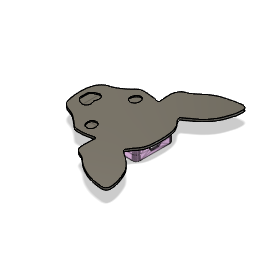
Case v4 (Autodesk Fusion 360 design; units mm, degrees)
Autodesk Fusion 360 part; units mm, degrees
mesh "Mesh1" [no effect]
sketch "Sketch1" plane through (0, 0, 0) normal (0, 1, 0) x (1, 0, 0)
  spline S0 degree 5 poles (79.7, 48.8) (79.719, 48.6987) (79.7514, 48.491) (79.7835, 48.1635) (79.7983, 47.6937) (79.7902, 47.047) (79.7751, 46.3439) (79.7599, 45.603) (79.7415, 44.8496) (79.7105, 44.1055) (79.6548, 43.3785) (79.5625, 42.6523) (79.4242, 41.8981) (79.2343, 41.0857) (78.9926, 40.1949) (78.7059, 39.2272) (78.3855, 38.1997) (78.0442, 37.1381) (77.6933, 36.0704) (77.3399, 35.0202) (76.9837, 33.9992) (76.6162, 33.0052) (76.2245, 32.0279) (75.7932, 31.0522) (75.3081, 30.0631) (74.7577, 29.0493) (74.1372, 28.0083) (73.4475, 26.9454) (72.6942, 25.8712) (71.8865, 24.8005) (71.0365, 23.75) (70.1577, 22.7363) (69.2645, 21.7746) (68.3706, 20.8762) (67.4886, 20.0487) (66.6282, 19.2945) (65.7956, 18.6106) (64.9922, 17.9877) (64.2136, 17.4094) (63.4483, 16.8517) (62.6821, 16.2893) (61.9016, 15.7016) (61.0986, 15.0793) (60.2738, 14.4301) (59.4412, 13.7868) (58.626, 13.1925) (57.8615, 12.684) (57.1871, 12.2757) (56.6448, 11.9441) (56.277, 11.6091) (56.116, 11.1755) (56.1708, 10.5839) (56.4188, 9.8471) (56.8189, 9.0183) (57.3225, 8.1658) (57.8852, 7.3451) (58.4778, 6.5734) (59.0828, 5.8405) (59.6904, 5.1182) (60.2951, 4.3704) (60.8923, 3.5627) (61.4748, 2.6725) (62.0334, 1.6874) (62.5584, 0.6036) (63.0405, -0.5757) (63.4715, -1.842) (63.846, -3.1831) (64.1621, -4.5843) (64.4206, -6.0301) (64.6252, -7.5046) (64.7808, -8.9924) (64.8936, -10.4799) (64.9703, -11.9557) (65.0169, -13.4121) (65.0389, -14.8453) (65.04, -16.2568) (65.0223, -17.6506) (64.9858, -19.0325) (64.9283, -20.4085) (64.8449, -21.783) (64.7281, -23.1575) (64.5673, -24.5293) (64.3484, -25.8898) (64.0567, -27.2263) (63.6793, -28.5249) (63.2076, -29.7715) (62.6403, -30.9546) (61.9852, -32.0673) (61.2629, -33.1089) (60.5082, -34.0874) (59.7625, -35.0146) (59.0668, -35.9023) (58.4531, -36.7574) (57.9381, -37.5785) (57.514, -38.3507) (57.1437, -39.0427) (56.7888, -39.6265) (56.4337, -40.094) (56.1169, -40.4782) (55.9432, -40.8613) (56.0142, -41.3227) (56.3554, -41.884) (56.9227, -42.515) (57.6412, -43.1657) (58.4327, -43.7883) (59.2513, -44.367) (60.0798, -44.9122) (60.9194, -45.4502) (61.7815, -46.0133) (62.6791, -46.6312) (63.617, -47.319) (64.5891, -48.0757) (65.5823, -48.8903) (66.5796, -49.7451) (67.5624, -50.6213) (68.5134, -51.5029) (69.4201, -52.3815) (70.2766, -53.2606) (71.083, -54.1521) (71.8431, -55.0725) (72.5629, -56.0393) (73.2493, -57.0672) (73.908, -58.165) (74.5421, -59.3304) (75.1517, -60.5514) (75.7351, -61.8097) (76.289, -63.0836) (76.8097, -64.3512) (77.294, -65.5936) (77.7391, -66.7979) (78.1445, -67.9606) (78.511, -69.0876) (78.84, -70.1896) (79.1328, -71.2793) (79.3893, -72.3679) (79.6075, -73.462) (79.7822, -74.5597) (79.9052, -75.6495) (79.9659, -76.714) (79.9523, -77.7308) (79.8515, -78.676) (79.651, -79.5255) (79.3392, -80.2577) (78.9071, -80.8561) (78.351, -81.3116) (77.674, -81.6255) (76.8884, -81.8117) (76.0116, -81.8922) (75.0626, -81.8922) (74.0586, -81.8357) (73.0105, -81.7401) (71.923, -81.6152) (70.7963, -81.4652) (69.6276, -81.2893) (68.413, -81.0833) (67.1491, -80.8408) (65.8342, -80.5541) (64.4698, -80.2157) (63.0597, -79.8186) (61.611, -79.3574) (60.1335, -78.8292) (58.6404, -78.2344) (57.148, -77.5774) (55.6761, -76.8675) (54.2482, -76.12) (52.889, -75.3539) (51.6218, -74.5894) (50.4661, -73.8459) (49.435, -73.1396) (48.5326, -72.4808) (47.752, -71.8723) (47.0713, -71.306) (46.4572, -70.7653) (45.8728, -70.232) (45.2832, -69.6907) (44.6638, -69.135) (44.0045, -68.5721) (43.3058, -68.0165) (42.5737, -67.4855) (41.8163, -66.994) (41.0385, -66.5495) (40.2417, -66.1497) (39.4275, -65.7856) (38.5995, -65.4415) (37.7661, -65.0972) (36.9437, -64.7285) (36.1534, -64.3102) (35.4181, -63.8185) (34.7592, -63.2338) (34.1931, -62.5432) (33.729, -61.7429) (33.3694, -60.8357) (33.1113, -59.8303) (32.9461, -58.7397) (32.8605, -57.58) (32.8372, -56.369) (32.8572, -55.1269) (32.9019, -53.8757) (32.9551, -52.6402) (33.0054, -51.4474) (33.0477, -50.327) (33.0862, -49.3112) (33.1287, -48.4278) (33.1813, -47.6907) (33.2433, -47.0941) (33.3012, -46.5995) (33.3258, -46.144) (33.2803, -45.6894) (33.1245, -45.2796) (32.838, -45.0016) (32.4755, -44.8703) (32.1398, -44.8181) (31.805, -44.8087) (31.3175, -44.855) (30.5696, -44.9693) (29.5634, -45.146) (28.365, -45.3694) (27.0805, -45.6165) (25.8227, -45.8622) (24.6834, -46.0835) (23.6982, -46.264) (22.8543, -46.3952) (22.1108, -46.4756) (21.4135, -46.5108) (20.7135, -46.5135) (19.9814, -46.5025) (19.2037, -46.4951) (18.3803, -46.5) (17.5215, -46.5088) (16.6451, -46.4914) (15.7717, -46.4081) (14.9204, -46.22) (14.1044, -45.8996) (13.3254, -45.4441) (12.575, -44.8733) (11.8395, -44.2198) (11.104, -43.5216) (10.3563, -42.8135) (9.5919, -42.1181) (8.8134, -41.4453) (8.0275, -40.7972) (7.2424, -40.1706) (6.4656, -39.5608) (5.7008, -38.9653) (4.9465, -38.3857) (4.1979, -37.8258) (3.4476, -37.291) (2.6872, -36.787) (1.9079, -36.3185) (1.1022, -35.8884) (0.2644, -35.4967) (-0.6087, -35.1391) (-1.5164, -34.807) (-2.4532, -34.4852) (-3.4094, -34.1535) (-4.3718, -33.7897) (-5.3247, -33.3723) (-6.2513, -32.8831) (-7.1342, -32.3101) (-7.9567, -31.6496) (-8.7041, -30.9033) (-9.3652, -30.0772) (-9.9331, -29.1799) (-10.4069, -28.2204) (-10.7931, -27.2066) (-11.1036, -26.1451) (-11.3536, -25.0408) (-11.5592, -23.8975) (-11.7349, -22.7174) (-11.8914, -21.5015) (-12.0333, -20.2492) (-12.16, -18.9596) (-12.2674, -17.6322) (-12.3489, -16.2679) (-12.3967, -14.8699) (-12.4034, -13.445) (-12.3627, -12.0041) (-12.2712, -10.5634) (-12.1273, -9.142) (-11.9309, -7.7602) (-11.6825, -6.4374) (-11.3825, -5.1897) (-11.0307, -4.0283) (-10.6255, -2.9572) (-10.1631, -1.971) (-9.6398, -1.0591) (-9.0533, -0.2097) (-8.4053, 0.5854) (-7.7029, 1.3276) (-6.9613, 2.0057) (-6.2025, 2.5971) (-5.4492, 3.0793) (-4.7184, 3.439) (-4.0167, 3.6808) (-3.3325, 3.8397) (-2.6411, 3.9728) (-1.9139, 4.1408) (-1.1273, 4.3941) (-0.2718, 4.7548) (0.6493, 5.2209) (1.6234, 5.7747) (2.6318, 6.39) (3.6529, 7.0395) (4.665, 7.7026) (5.6494, 8.3694) (6.5901, 9.0365) (7.4756, 9.7051) (8.2993, 10.3779) (9.0603, 11.0569) (9.7649, 11.7402) (10.4259, 12.4209) (11.0615, 13.0884) (11.6936, 13.7292) (12.3466, 14.3276) (13.0462, 14.8661) (13.8171, 15.3277) (14.6807, 15.6975) (15.6529, 15.9655) (16.7413, 16.1284) (17.9426, 16.1926) (19.243, 16.1724) (20.6205, 16.0873) (22.0464, 15.9583) (23.4868, 15.8057) (24.9046, 15.6459) (26.2614, 15.4886) (27.5183, 15.3328) (28.6412, 15.1715) (29.6053, 14.9976) (30.4017, 14.8101) (31.0401, 14.6197) (31.5593, 14.4564) (32.0179, 14.3687) (32.4563, 14.4031) (32.8494, 14.5822) (33.1244, 14.9053) (33.2471, 15.3733) (33.2474, 15.9939) (33.1791, 16.7718) (33.0898, 17.6996) (33.0018, 18.7535) (32.9234, 19.9011) (32.8536, 21.1057) (32.789, 22.3319) (32.7295, 23.5506) (32.6863, 24.7456) (32.6806, 25.9121) (32.738, 27.0512) (32.8842, 28.1659) (33.1401, 29.2558) (33.5175, 30.3134) (34.0136, 31.3181) (34.6121, 32.2394) (35.2891, 33.0464) (36.0178, 33.7154) (36.7729, 34.237) (37.5359, 34.6256) (38.2984, 34.9229) (39.0589, 35.1834) (39.8212, 35.4638) (40.5917, 35.8111) (41.378, 36.25) (42.1871, 36.7866) (43.0251, 37.4139) (43.896, 38.1159) (44.8012, 38.8726) (45.7384, 39.6653) (46.7022, 40.4774) (47.6866, 41.2944) (48.6859, 42.1039) (49.6968, 42.8958) (50.7197, 43.6621) (51.7606, 44.3973) (52.832, 45.098) (53.9494, 45.7628) (55.1293, 46.3915) (56.3853, 46.9846) (57.7261, 47.5433) (59.1523, 48.0682) (60.6535, 48.5596) (62.206, 49.0166) (63.7773, 49.4378) (65.3304, 49.8216) (66.8273, 50.1665) (68.2335, 50.4717) (69.5221, 50.7374) (70.6776, 50.9653) (71.7008, 51.1588) (72.6095, 51.3232) (73.4309, 51.4621) (74.1944, 51.5753) (74.925, 51.6566) (75.6357, 51.6895) (76.3257, 51.6523) (76.9846, 51.529) (77.5943, 51.3184) (78.1315, 51.0447) (78.5772, 50.7396) (78.926, 50.4252) (79.1962, 50.0932) (79.4146, 49.7205) (79.5553, 49.3789) (79.6375, 49.0986) (79.681, 48.9013) (79.7, 48.8) knots 0 0 0 0 0 0 0.0025 0.005 0.0075 0.01 0.0125 0.015 0.0175 0.02 0.0225 0.025 0.0275 0.03 0.0325 0.035 0.0375 0.04 0.0425 0.045 0.0475 0.05 0.0525 0.055 0.0575 0.06 0.0625 0.065 0.0675 0.07 0.0725 0.075 0.0775 0.08 0.0825 0.085 0.0875 0.09 0.0925 0.095 0.0975 0.1 0.1025 0.105 0.1075 0.11 0.1125 0.115 0.1175 0.12 0.1225 0.125 0.1275 0.13 0.1325 0.135 0.1375 0.14 0.1425 0.145 0.1475 0.15 0.1525 0.155 0.1575 0.16 0.1625 0.165 0.1675 0.17 0.1725 0.175 0.1775 0.18 0.1825 0.185 0.1875 0.19 0.1925 0.195 0.1975 0.2 0.2025 0.205 0.2075 0.21 0.2125 0.215 0.2175 0.22 0.2225 0.225 0.2275 0.23 0.2325 0.235 0.2375 0.24 0.2425 0.245 0.2475 0.25 0.2525 0.255 0.2575 0.26 0.2625 0.265 0.2675 0.27 0.2725 0.275 0.2775 0.28 0.2825 0.285 0.2875 0.29 0.2925 0.295 0.2975 0.3 0.3025 0.305 0.3075 0.31 0.3125 0.315 0.3175 0.32 0.3225 0.325 0.3275 0.33 0.3325 0.335 0.3375 0.34 0.3425 0.345 0.3475 0.35 0.3525 0.355 0.3575 0.36 0.3625 0.365 0.3675 0.37 0.3725 0.375 0.3775 0.38 0.3825 0.385 0.3875 0.39 0.3925 0.395 0.3975 0.4 0.4025 0.405 0.4075 0.41 0.4125 0.415 0.4175 0.42 0.4225 0.425 0.4275 0.43 0.4325 0.435 0.4375 0.44 0.4425 0.445 0.4475 0.45 0.4525 0.455 0.4575 0.46 0.4625 0.465 0.4675 0.47 0.4725 0.475 0.4775 0.48 0.4825 0.485 0.4875 0.49 0.4925 0.495 0.4975 0.5 0.5025 0.505 0.5075 0.51 0.5125 0.515 0.5175 0.52 0.5225 0.525 0.5275 0.53 0.5325 0.535 0.5375 0.54 0.5425 0.545 0.5475 0.55 0.5525 0.555 0.5575 0.56 0.5625 0.565 0.5675 0.57 0.5725 0.575 0.5775 0.58 0.5825 0.585 0.5875 0.59 0.5925 0.595 0.5975 0.6 0.6025 0.605 0.6075 0.61 0.6125 0.615 0.6175 0.62 0.6225 0.625 0.6275 0.63 0.6325 0.635 0.6375 0.64 0.6425 0.645 0.6475 0.65 0.6525 0.655 0.6575 0.66 0.6625 0.665 0.6675 0.67 0.6725 0.675 0.6775 0.68 0.6825 0.685 0.6875 0.69 0.6925 0.695 0.6975 0.7 0.7025 0.705 0.7075 0.71 0.7125 0.715 0.7175 0.72 0.7225 0.725 0.7275 0.73 0.7325 0.735 0.7375 0.74 0.7425 0.745 0.7475 0.75 0.7525 0.755 0.7575 0.76 0.7625 0.765 0.7675 0.77 0.7725 0.775 0.7775 0.78 0.7825 0.785 0.7875 0.79 0.7925 0.795 0.7975 0.8 0.8025 0.805 0.8075 0.81 0.8125 0.815 0.8175 0.82 0.8225 0.825 0.8275 0.83 0.8325 0.835 0.8375 0.84 0.8425 0.845 0.8475 0.85 0.8525 0.855 0.8575 0.86 0.8625 0.865 0.8675 0.87 0.8725 0.875 0.8775 0.88 0.8825 0.885 0.8875 0.89 0.8925 0.895 0.8975 0.9 0.9025 0.905 0.9075 0.91 0.9125 0.915 0.9175 0.92 0.9225 0.925 0.9275 0.93 0.9325 0.935 0.9375 0.94 0.9425 0.945 0.9475 0.95 0.9525 0.955 0.9575 0.96 0.9625 0.965 0.9675 0.97 0.9725 0.975 0.9775 0.98 0.9825 0.985 0.9875 0.99 0.9925 0.995 0.9975 1 1 1 1 1 1
  point P0 (79.7869, 46.9408)
  point P1 (79.7048, 44.1167)
  point P2 (79.2122, 41.0299)
  point P3 (77.5, 35.5)
  point P4 (75.193, 29.8677)
  point P5 (70.2659, 22.8745)
  point P6 (65, 18)
  point P7 (61, 15)
  point P8 (57.1735, 12.2655)
  point P9 (56.1802, 11.2125)
  point P10 (57.3126, 8.2126)
  point P11 (60.2997, 4.347)
  point P12 (63.5, -2)
  point P13 (65, -13)
  point P14 (64.7162, -23.1652)
  point P15 (62, -32)
  point P16 (58, -37.5)
  point P17 (56.5, -40)
  point P18 (56, -41)
  point P19 (57.7878, -43.2659)
  point P20 (62.2077, -46.3112)
  point P21 (68.5, -51.5)
  point P22 (73.5, -57.5)
  point P23 (77.4744, -66.0904)
  point P24 (79.5, -72.9496)
  point P25 (79.8271, -78.649)
  point P26 (78.336, -81.2667)
  point P27 (74.6579, -81.8632)
  point P28 (68, -81)
  point P29 (57.0626, -77.5224)
  point P30 (48.2484, -72.2537)
  point P31 (45.3656, -69.7685)
  point P32 (42.2508, -67.2833)
  point P33 (38.5097, -65.4045)
  point P34 (34.9376, -63.3633)
  point P35 (33, -59)
  point P36 (33.0058, -51.4078)
  point P37 (33.2245, -47.289)
  point P38 (33.3, -46)
  point P39 (32.9569, -45.1468)
  point P40 (32.3074, -44.8515)
  point P41 (31.466, -44.8466)
  point P42 (25.5907, -45.9068)
  point P43 (21.5, -46.5)
  point P44 (18.5, -46.5)
  point P45 (14.6259, -46.0847)
  point P46 (10.8622, -43.2937)
  point P47 (6.7439, -39.7801)
  point P48 (3, -37)
  point P49 (-1, -35)
  point P50 (-6, -33)
  point P51 (-10, -29)
  point P52 (-11.7363, -22.6636)
  point P53 (-12.3921, -13.4829)
  point P54 (-11, -4)
  point P55 (-8, 1)
  point P56 (-4.5, 3.5)
  point P57 (-1.7755, 4.1976)
  point P58 (3.2385, 6.7787)
  point P59 (8.6974, 10.7403)
  point P60 (12, 14)
  point P61 (16, 16)
  point P62 (25.2363, 15.6066)
  point P63 (30.8294, 14.6801)
  point P64 (32.2, 14.4)
  point P65 (33, 14.8)
  point P66 (33.2, 16.5)
  point P67 (32.769, 22.762)
  point P68 (33.2893, 29.6228)
  point P69 (36.5734, 34.0774)
  point P70 (39.89, 35.5081)
  point P71 (44.117, 38.3045)
  point P72 (50.5226, 43.507)
  point P73 (59, 48)
  point P74 (70.2921, 50.888)
  point P75 (74.4866, 51.6033)
  point P76 (77, 51.5)
  point P77 (78.6, 50.7)
  point P78 (79.3, 49.9)
extrude "Extrude1" add sketch "Sketch1" along normal blind 2 from surface at 17
sketch "Sketch2" plane through (0, 19, 0) normal (0, 1, 0) x (-1, 0, 0)
  spline S0 degree 5 poles (-79.7, -48.8) (-79.681, -48.9013) (-79.6375, -49.0986) (-79.5553, -49.3789) (-79.4146, -49.7205) (-79.1962, -50.0932) (-78.926, -50.4252) (-78.5772, -50.7396) (-78.1315, -51.0447) (-77.5943, -51.3184) (-76.9846, -51.529) (-76.3257, -51.6523) (-75.6357, -51.6895) (-74.925, -51.6566) (-74.1944, -51.5753) (-73.4309, -51.4621) (-72.6095, -51.3232) (-71.7008, -51.1588) (-70.6776, -50.9653) (-69.5221, -50.7374) (-68.2335, -50.4717) (-66.8273, -50.1665) (-65.3304, -49.8216) (-63.7773, -49.4378) (-62.206, -49.0166) (-60.6535, -48.5596) (-59.1523, -48.0682) (-57.7261, -47.5433) (-56.3853, -46.9846) (-55.1293, -46.3915) (-53.9494, -45.7628) (-52.832, -45.098) (-51.7606, -44.3973) (-50.7197, -43.6621) (-49.6968, -42.8958) (-48.6859, -42.1039) (-47.6866, -41.2944) (-46.7022, -40.4774) (-45.7384, -39.6653) (-44.8012, -38.8726) (-43.896, -38.1159) (-43.0251, -37.4139) (-42.1871, -36.7866) (-41.378, -36.25) (-40.5917, -35.8111) (-39.8212, -35.4638) (-39.0589, -35.1834) (-38.2984, -34.9229) (-37.5359, -34.6256) (-36.7729, -34.237) (-36.0178, -33.7154) (-35.2891, -33.0464) (-34.6121, -32.2394) (-34.0136, -31.3181) (-33.5175, -30.3134) (-33.1401, -29.2558) (-32.8842, -28.1659) (-32.738, -27.0512) (-32.6806, -25.9121) (-32.6863, -24.7456) (-32.7295, -23.5506) (-32.789, -22.3319) (-32.8536, -21.1057) (-32.9234, -19.9011) (-33.0018, -18.7535) (-33.0898, -17.6996) (-33.1791, -16.7718) (-33.2474, -15.9939) (-33.2471, -15.3733) (-33.1244, -14.9053) (-32.8494, -14.5822) (-32.4563, -14.4031) (-32.0179, -14.3687) (-31.5593, -14.4564) (-31.0401, -14.6197) (-30.4017, -14.8101) (-29.6053, -14.9976) (-28.6412, -15.1715) (-27.5183, -15.3328) (-26.2614, -15.4886) (-24.9046, -15.6459) (-23.4868, -15.8057) (-22.0464, -15.9583) (-20.6205, -16.0873) (-19.243, -16.1724) (-17.9426, -16.1926) (-16.7413, -16.1284) (-15.6529, -15.9655) (-14.6807, -15.6975) (-13.8171, -15.3277) (-13.0462, -14.8661) (-12.3466, -14.3276) (-11.6936, -13.7292) (-11.0615, -13.0884) (-10.4259, -12.4209) (-9.7649, -11.7402) (-9.0603, -11.0569) (-8.2993, -10.3779) (-7.4756, -9.7051) (-6.5901, -9.0365) (-5.6494, -8.3694) (-4.665, -7.7026) (-3.6529, -7.0395) (-2.6318, -6.39) (-1.6234, -5.7747) (-0.6493, -5.2209) (0.2718, -4.7548) (1.1273, -4.3941) (1.9139, -4.1408) (2.6411, -3.9728) (3.3325, -3.8397) (4.0167, -3.6808) (4.7184, -3.439) (5.4492, -3.0793) (6.2025, -2.5971) (6.9613, -2.0057) (7.7029, -1.3276) (8.4053, -0.5854) (9.0533, 0.2097) (9.6398, 1.0591) (10.1631, 1.971) (10.6255, 2.9572) (11.0307, 4.0283) (11.3825, 5.1897) (11.6825, 6.4374) (11.9309, 7.7602) (12.1273, 9.142) (12.2712, 10.5634) (12.3627, 12.0041) (12.4034, 13.445) (12.3967, 14.8699) (12.3489, 16.2679) (12.2674, 17.6322) (12.16, 18.9596) (12.0333, 20.2492) (11.8914, 21.5015) (11.7349, 22.7174) (11.5592, 23.8975) (11.3536, 25.0408) (11.1036, 26.1451) (10.7931, 27.2066) (10.4069, 28.2204) (9.9331, 29.1799) (9.3652, 30.0772) (8.7041, 30.9033) (7.9567, 31.6496) (7.1342, 32.3101) (6.2513, 32.8831) (5.3247, 33.3723) (4.3718, 33.7897) (3.4094, 34.1535) (2.4532, 34.4852) (1.5164, 34.807) (0.6087, 35.1391) (-0.2644, 35.4967) (-1.1022, 35.8884) (-1.9079, 36.3185) (-2.6872, 36.787) (-3.4476, 37.291) (-4.1979, 37.8258) (-4.9465, 38.3857) (-5.7008, 38.9653) (-6.4656, 39.5608) (-7.2424, 40.1706) (-8.0275, 40.7972) (-8.8134, 41.4453) (-9.5919, 42.1181) (-10.3563, 42.8135) (-11.104, 43.5216) (-11.8395, 44.2198) (-12.575, 44.8733) (-13.3254, 45.4441) (-14.1044, 45.8996) (-14.9204, 46.22) (-15.7717, 46.4081) (-16.6451, 46.4914) (-17.5215, 46.5088) (-18.3803, 46.5) (-19.2037, 46.4951) (-19.9814, 46.5025) (-20.7135, 46.5135) (-21.4135, 46.5108) (-22.1108, 46.4756) (-22.8543, 46.3952) (-23.6982, 46.264) (-24.6834, 46.0835) (-25.8227, 45.8622) (-27.0805, 45.6165) (-28.365, 45.3694) (-29.5634, 45.146) (-30.5696, 44.9693) (-31.3175, 44.855) (-31.805, 44.8087) (-32.1398, 44.8181) (-32.4755, 44.8703) (-32.838, 45.0016) (-33.1245, 45.2796) (-33.2803, 45.6894) (-33.3258, 46.144) (-33.3012, 46.5995) (-33.2433, 47.0941) (-33.1813, 47.6907) (-33.1287, 48.4278) (-33.0862, 49.3112) (-33.0477, 50.327) (-33.0054, 51.4474) (-32.9551, 52.6402) (-32.9019, 53.8757) (-32.8572, 55.1269) (-32.8372, 56.369) (-32.8605, 57.58) (-32.9461, 58.7397) (-33.1113, 59.8303) (-33.3694, 60.8357) (-33.729, 61.7429) (-34.1931, 62.5432) (-34.7592, 63.2338) (-35.4181, 63.8185) (-36.1534, 64.3102) (-36.9437, 64.7285) (-37.7661, 65.0972) (-38.5995, 65.4415) (-39.4275, 65.7856) (-40.2417, 66.1497) (-41.0385, 66.5495) (-41.8163, 66.994) (-42.5737, 67.4855) (-43.3058, 68.0165) (-44.0045, 68.5721) (-44.6638, 69.135) (-45.2832, 69.6907) (-45.8728, 70.232) (-46.4572, 70.7653) (-47.0713, 71.306) (-47.752, 71.8723) (-48.5326, 72.4808) (-49.435, 73.1396) (-50.4661, 73.8459) (-51.6218, 74.5894) (-52.889, 75.3539) (-54.2482, 76.12) (-55.6761, 76.8675) (-57.148, 77.5774) (-58.6404, 78.2344) (-60.1335, 78.8292) (-61.611, 79.3574) (-63.0597, 79.8186) (-64.4698, 80.2157) (-65.8342, 80.5541) (-67.1491, 80.8408) (-68.413, 81.0833) (-69.6276, 81.2893) (-70.7963, 81.4652) (-71.923, 81.6152) (-73.0105, 81.7401) (-74.0586, 81.8357) (-75.0626, 81.8922) (-76.0116, 81.8922) (-76.8884, 81.8117) (-77.674, 81.6255) (-78.351, 81.3116) (-78.9071, 80.8561) (-79.3392, 80.2577) (-79.651, 79.5255) (-79.8515, 78.676) (-79.9523, 77.7308) (-79.9659, 76.714) (-79.9052, 75.6495) (-79.7822, 74.5597) (-79.6075, 73.462) (-79.3893, 72.3679) (-79.1328, 71.2793) (-78.84, 70.1896) (-78.511, 69.0876) (-78.1445, 67.9606) (-77.7391, 66.7979) (-77.294, 65.5936) (-76.8097, 64.3512) (-76.289, 63.0836) (-75.7351, 61.8097) (-75.1517, 60.5514) (-74.5421, 59.3304) (-73.908, 58.165) (-73.2493, 57.0672) (-72.5629, 56.0393) (-71.8431, 55.0725) (-71.083, 54.1521) (-70.2766, 53.2606) (-69.4201, 52.3815) (-68.5134, 51.5029) (-67.5624, 50.6213) (-66.5796, 49.7451) (-65.5823, 48.8903) (-64.5891, 48.0757) (-63.617, 47.319) (-62.6791, 46.6312) (-61.7815, 46.0133) (-60.9194, 45.4502) (-60.0798, 44.9122) (-59.2513, 44.367) (-58.4327, 43.7883) (-57.6412, 43.1657) (-56.9227, 42.515) (-56.3554, 41.884) (-56.0142, 41.3227) (-55.9432, 40.8613) (-56.1169, 40.4782) (-56.4337, 40.094) (-56.7888, 39.6265) (-57.1437, 39.0427) (-57.514, 38.3507) (-57.9381, 37.5785) (-58.4531, 36.7574) (-59.0668, 35.9023) (-59.7625, 35.0146) (-60.5082, 34.0874) (-61.2629, 33.1089) (-61.9852, 32.0673) (-62.6403, 30.9546) (-63.2076, 29.7715) (-63.6793, 28.5249) (-64.0567, 27.2263) (-64.3484, 25.8898) (-64.5673, 24.5293) (-64.7281, 23.1575) (-64.8449, 21.783) (-64.9283, 20.4085) (-64.9858, 19.0325) (-65.0223, 17.6506) (-65.04, 16.2568) (-65.0389, 14.8453) (-65.0169, 13.4121) (-64.9703, 11.9557) (-64.8936, 10.4799) (-64.7808, 8.9924) (-64.6252, 7.5046) (-64.4206, 6.0301) (-64.1621, 4.5843) (-63.846, 3.1831) (-63.4715, 1.842) (-63.0405, 0.5757) (-62.5584, -0.6036) (-62.0334, -1.6874) (-61.4748, -2.6725) (-60.8923, -3.5627) (-60.2951, -4.3704) (-59.6904, -5.1182) (-59.0828, -5.8405) (-58.4778, -6.5734) (-57.8852, -7.3451) (-57.3225, -8.1658) (-56.8189, -9.0183) (-56.4188, -9.8471) (-56.1708, -10.5839) (-56.116, -11.1755) (-56.277, -11.6091) (-56.6448, -11.9441) (-57.1871, -12.2757) (-57.8615, -12.684) (-58.626, -13.1925) (-59.4412, -13.7868) (-60.2738, -14.4301) (-61.0986, -15.0793) (-61.9016, -15.7016) (-62.6821, -16.2893) (-63.4483, -16.8517) (-64.2136, -17.4094) (-64.9922, -17.9877) (-65.7956, -18.6106) (-66.6282, -19.2945) (-67.4886, -20.0487) (-68.3706, -20.8762) (-69.2645, -21.7746) (-70.1577, -22.7363) (-71.0365, -23.75) (-71.8865, -24.8005) (-72.6942, -25.8712) (-73.4475, -26.9454) (-74.1372, -28.0083) (-74.7577, -29.0493) (-75.3081, -30.0631) (-75.7932, -31.0522) (-76.2245, -32.0279) (-76.6162, -33.0052) (-76.9837, -33.9992) (-77.3399, -35.0202) (-77.6933, -36.0704) (-78.0442, -37.1381) (-78.3855, -38.1997) (-78.7059, -39.2272) (-78.9926, -40.1949) (-79.2343, -41.0857) (-79.4242, -41.8981) (-79.5625, -42.6523) (-79.6548, -43.3785) (-79.7105, -44.1055) (-79.7415, -44.8496) (-79.7599, -45.603) (-79.7751, -46.3439) (-79.7902, -47.047) (-79.7983, -47.6937) (-79.7835, -48.1635) (-79.7514, -48.491) (-79.719, -48.6987) (-79.7, -48.8) knots -1 -1 -1 -1 -1 -1 -0.9975 -0.995 -0.9925 -0.99 -0.9875 -0.985 -0.9825 -0.98 -0.9775 -0.975 -0.9725 -0.97 -0.9675 -0.965 -0.9625 -0.96 -0.9575 -0.955 -0.9525 -0.95 -0.9475 -0.945 -0.9425 -0.94 -0.9375 -0.935 -0.9325 -0.93 -0.9275 -0.925 -0.9225 -0.92 -0.9175 -0.915 -0.9125 -0.91 -0.9075 -0.905 -0.9025 -0.9 -0.8975 -0.895 -0.8925 -0.89 -0.8875 -0.885 -0.8825 -0.88 -0.8775 -0.875 -0.8725 -0.87 -0.8675 -0.865 -0.8625 -0.86 -0.8575 -0.855 -0.8525 -0.85 -0.8475 -0.845 -0.8425 -0.84 -0.8375 -0.835 -0.8325 -0.83 -0.8275 -0.825 -0.8225 -0.82 -0.8175 -0.815 -0.8125 -0.81 -0.8075 -0.805 -0.8025 -0.8 -0.7975 -0.795 -0.7925 -0.79 -0.7875 -0.785 -0.7825 -0.78 -0.7775 -0.775 -0.7725 -0.77 -0.7675 -0.765 -0.7625 -0.76 -0.7575 -0.755 -0.7525 -0.75 -0.7475 -0.745 -0.7425 -0.74 -0.7375 -0.735 -0.7325 -0.73 -0.7275 -0.725 -0.7225 -0.72 -0.7175 -0.715 -0.7125 -0.71 -0.7075 -0.705 -0.7025 -0.7 -0.6975 -0.695 -0.6925 -0.69 -0.6875 -0.685 -0.6825 -0.68 -0.6775 -0.675 -0.6725 -0.67 -0.6675 -0.665 -0.6625 -0.66 -0.6575 -0.655 -0.6525 -0.65 -0.6475 -0.645 -0.6425 -0.64 -0.6375 -0.635 -0.6325 -0.63 -0.6275 -0.625 -0.6225 -0.62 -0.6175 -0.615 -0.6125 -0.61 -0.6075 -0.605 -0.6025 -0.6 -0.5975 -0.595 -0.5925 -0.59 -0.5875 -0.585 -0.5825 -0.58 -0.5775 -0.575 -0.5725 -0.57 -0.5675 -0.565 -0.5625 -0.56 -0.5575 -0.555 -0.5525 -0.55 -0.5475 -0.545 -0.5425 -0.54 -0.5375 -0.535 -0.5325 -0.53 -0.5275 -0.525 -0.5225 -0.52 -0.5175 -0.515 -0.5125 -0.51 -0.5075 -0.505 -0.5025 -0.5 -0.4975 -0.495 -0.4925 -0.49 -0.4875 -0.485 -0.4825 -0.48 -0.4775 -0.475 -0.4725 -0.47 -0.4675 -0.465 -0.4625 -0.46 -0.4575 -0.455 -0.4525 -0.45 -0.4475 -0.445 -0.4425 -0.44 -0.4375 -0.435 -0.4325 -0.43 -0.4275 -0.425 -0.4225 -0.42 -0.4175 -0.415 -0.4125 -0.41 -0.4075 -0.405 -0.4025 -0.4 -0.3975 -0.395 -0.3925 -0.39 -0.3875 -0.385 -0.3825 -0.38 -0.3775 -0.375 -0.3725 -0.37 -0.3675 -0.365 -0.3625 -0.36 -0.3575 -0.355 -0.3525 -0.35 -0.3475 -0.345 -0.3425 -0.34 -0.3375 -0.335 -0.3325 -0.33 -0.3275 -0.325 -0.3225 -0.32 -0.3175 -0.315 -0.3125 -0.31 -0.3075 -0.305 -0.3025 -0.3 -0.2975 -0.295 -0.2925 -0.29 -0.2875 -0.285 -0.2825 -0.28 -0.2775 -0.275 -0.2725 -0.27 -0.2675 -0.265 -0.2625 -0.26 -0.2575 -0.255 -0.2525 -0.25 -0.2475 -0.245 -0.2425 -0.24 -0.2375 -0.235 -0.2325 -0.23 -0.2275 -0.225 -0.2225 -0.22 -0.2175 -0.215 -0.2125 -0.21 -0.2075 -0.205 -0.2025 -0.2 -0.1975 -0.195 -0.1925 -0.19 -0.1875 -0.185 -0.1825 -0.18 -0.1775 -0.175 -0.1725 -0.17 -0.1675 -0.165 -0.1625 -0.16 -0.1575 -0.155 -0.1525 -0.15 -0.1475 -0.145 -0.1425 -0.14 -0.1375 -0.135 -0.1325 -0.13 -0.1275 -0.125 -0.1225 -0.12 -0.1175 -0.115 -0.1125 -0.11 -0.1075 -0.105 -0.1025 -0.1 -0.0975 -0.095 -0.0925 -0.09 -0.0875 -0.085 -0.0825 -0.08 -0.0775 -0.075 -0.0725 -0.07 -0.0675 -0.065 -0.0625 -0.06 -0.0575 -0.055 -0.0525 -0.05 -0.0475 -0.045 -0.0425 -0.04 -0.0375 -0.035 -0.0325 -0.03 -0.0275 -0.025 -0.0225 -0.02 -0.0175 -0.015 -0.0125 -0.01 -0.0075 -0.005 -0.0025 0 0 0 0 0 0
  spline S1 degree 5 poles (-21.9, 31.6) (-21.9594, 31.6337) (-22.0768, 31.7044) (-22.2495, 31.8196) (-22.4754, 31.991) (-22.748, 32.2339) (-23.0047, 32.5042) (-23.24, 32.7995) (-23.4516, 33.117) (-23.6388, 33.4551) (-23.8022, 33.8155) (-23.9429, 34.205) (-24.0616, 34.6344) (-24.1576, 35.1137) (-24.2276, 35.6486) (-24.2643, 36.2363) (-24.2563, 36.8627) (-24.1902, 37.5067) (-24.0527, 38.1431) (-23.8329, 38.7459) (-23.5245, 39.2917) (-23.1279, 39.7632) (-22.6508, 40.1499) (-22.1056, 40.4459) (-21.5086, 40.6485) (-20.8779, 40.7571) (-20.2323, 40.7707) (-19.5893, 40.6877) (-18.9654, 40.5061) (-18.3753, 40.2248) (-17.8319, 39.8452) (-17.3457, 39.3713) (-16.9248, 38.8118) (-16.5744, 38.18) (-16.298, 37.4928) (-16.0979, 36.7694) (-15.9759, 36.0302) (-15.9344, 35.2961) (-15.9763, 34.5865) (-16.1068, 33.9192) (-16.3307, 33.3091) (-16.6506, 32.7684) (-17.0644, 32.3059) (-17.563, 31.9269) (-18.1282, 31.6325) (-18.7308, 31.4196) (-19.3371, 31.282) (-19.9141, 31.2118) (-20.4352, 31.2001) (-20.8855, 31.2384) (-21.2685, 31.3197) (-21.5343, 31.4151) (-21.7203, 31.5019) (-21.8406, 31.5663) (-21.9, 31.6) knots 0 0 0 0 0 0 0.02 0.04 0.06 0.08 0.1 0.12 0.14 0.16 0.18 0.2 0.22 0.24 0.26 0.28 0.3 0.32 0.34 0.36 0.38 0.4 0.42 0.44 0.46 0.48 0.5 0.52 0.54 0.56 0.58 0.6 0.62 0.64 0.66 0.68 0.7 0.72 0.74 0.76 0.78 0.8 0.82 0.84 0.86 0.88 0.9 0.92 0.94 0.96 0.98 1 1 1 1 1 1
  spline S2 degree 5 poles (-23.5098, -8.5144) (-23.5711, -8.4113) (-23.6861, -8.2053) (-23.8364, -7.8978) (-23.9955, -7.4925) (-24.1361, -6.9835) (-24.2278, -6.4565) (-24.2746, -5.8972) (-24.2708, -5.3011) (-24.203, -4.6731) (-24.055, -4.0256) (-23.8113, -3.377) (-23.4611, -2.7501) (-23.0012, -2.1707) (-22.4358, -1.665) (-21.7761, -1.2585) (-21.0401, -0.9732) (-20.2528, -0.8259) (-19.4458, -0.8263) (-18.6543, -0.9769) (-17.914, -1.274) (-17.2579, -1.7079) (-16.7133, -2.2631) (-16.2978, -2.919) (-16.0191, -3.6506) (-15.8773, -4.431) (-15.8667, -5.2333) (-15.9779, -6.0324) (-16.1995, -6.8072) (-16.5204, -7.5423) (-16.929, -8.2261) (-17.4132, -8.8489) (-17.9602, -9.4002) (-18.5564, -9.8674) (-19.1867, -10.2328) (-19.8348, -10.4748) (-20.484, -10.5744) (-21.1172, -10.5197) (-21.7182, -10.3115) (-22.2716, -9.9697) (-22.7638, -9.5298) (-23.1005, -9.1316) (-23.3185, -8.8236) (-23.4486, -8.6174) (-23.5098, -8.5144) knots 0 0 0 0 0 0 0.025 0.05 0.075 0.1 0.125 0.15 0.175 0.2 0.225 0.25 0.275 0.3 0.325 0.35 0.375 0.4 0.425 0.45 0.475 0.5 0.525 0.55 0.575 0.6 0.625 0.65 0.675 0.7 0.725 0.75 0.775 0.8 0.825 0.85 0.875 0.9 0.925 0.95 0.975 1 1 1 1 1 1
  spline S3 degree 5 poles (7.7509, 15.4792) (7.7463, 15.3221) (7.7417, 15.0047) (7.7496, 14.5195) (7.7839, 13.8566) (7.8253, 13.0186) (7.8096, 12.1943) (7.6819, 11.4079) (7.4001, 10.6803) (6.9519, 10.0235) (6.3583, 9.4392) (5.6599, 8.9232) (4.9077, 8.4683) (4.1512, 8.0677) (3.4294, 7.7179) (2.7576, 7.4228) (2.1321, 7.1923) (1.5389, 7.0385) (0.9612, 6.9741) (0.387, 7.0089) (-0.1833, 7.1476) (-0.7403, 7.3909) (-1.2679, 7.7361) (-1.7466, 8.1784) (-2.1556, 8.7117) (-2.476, 9.3274) (-2.6935, 10.0133) (-2.8012, 10.7525) (-2.8025, 11.5212) (-2.7135, 12.2889) (-2.5593, 13.0242) (-2.371, 13.7005) (-2.1831, 14.3021) (-2.0297, 14.8298) (-1.942, 15.3055) (-1.9416, 15.7608) (-2.0354, 16.2269) (-2.2078, 16.7226) (-2.4228, 17.2519) (-2.6356, 17.8113) (-2.8018, 18.3949) (-2.889, 19.0012) (-2.8796, 19.6335) (-2.7646, 20.2932) (-2.5396, 20.9739) (-2.1998, 21.6562) (-1.735, 22.3015) (-1.135, 22.8604) (-0.3933, 23.2809) (0.487, 23.5172) (1.4893, 23.5377) (2.5772, 23.3352) (3.6958, 22.9278) (4.7815, 22.3504) (5.7696, 21.6483) (6.6022, 20.8706) (7.2364, 20.0633) (7.652, 19.2629) (7.8612, 18.4886) (7.9106, 17.7391) (7.864, 17.0013) (7.8034, 16.4054) (7.7693, 15.9476) (7.7555, 15.6363) (7.7509, 15.4792) knots 0 0 0 0 0 0 0.01666667 0.03333333 0.05 0.06666667 0.08333333 0.1 0.11666667 0.13333333 0.15 0.16666667 0.18333333 0.2 0.21666667 0.23333333 0.25 0.26666667 0.28333333 0.3 0.31666667 0.33333333 0.35 0.36666667 0.38333333 0.4 0.41666667 0.43333333 0.45 0.46666667 0.48333333 0.5 0.51666667 0.53333333 0.55 0.56666667 0.58333333 0.6 0.61666667 0.63333333 0.65 0.66666667 0.68333333 0.7 0.71666667 0.73333333 0.75 0.76666667 0.78333333 0.8 0.81666667 0.83333333 0.85 0.86666667 0.88333333 0.9 0.91666667 0.93333333 0.95 0.96666667 0.98333333 1 1 1 1 1 1
  point P0 (-22.9, 32.4)
  point P1 (-23.7, 33.6)
  point P2 (-24.2068, 35.5385)
  point P3 (-23.6898, 38.9712)
  point P4 (-20.9189, 40.7288)
  point P5 (-17.5, 39.5)
  point P6 (-15.9561, 35.2077)
  point P7 (-17.5, 32)
  point P8 (-20.526, 31.2167)
  point P9 (-24.2266, -6.364)
  point P10 (-23.8512, -3.531)
  point P11 (-21, -1)
  point P12 (-17, -2)
  point P13 (-16, -6)
  point P14 (-18.2875, -9.6408)
  point P15 (-21.3253, -10.4258)
  point P16 (7.5, 11)
  point P17 (4, 8)
  point P18 (1, 7)
  point P19 (-1.3163, 7.809)
  point P20 (-2.766, 10.6557)
  point P21 (-2.2125, 14.214)
  point P22 (-2, 16)
  point P23 (-2.7133, 18.115)
  point P24 (-2.5, 21)
  point P25 (1, 23.5)
  point P26 (7.5, 19.5)
extrude "Extrude2" cut sketch "Sketch2" against normal blind 1 contours S1 | S2 | S3
